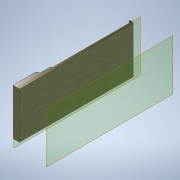
# Autodesk Inventor part: ShipDesign-ver3-1111-2021
Saved by Autodesk Inventor 2021 (Build 250183000, 183)
## iProperties
Created: 2021-02-04
Part Number: ShipDesign-ver3-1111-2021
Material: Wood (Oak)
Document SubType Name: Modeling
Designer: CMurray
Density: 0.76 g/cm^3
Appearance: Wood - Vertical White
Author: CMurray
Autodesk Inventor part; units mm, degrees
ref_plane "YZ Plane" through (0, 0, 0) normal (1, 0, 0) x (0, 1, 0)
ref_plane "XZ Plane" through (0, 0, 0) normal (0, 1, 0) x (-1, 0, 0)
ref_plane "XY Plane" through (0, 0, 0) normal (0, 0, 1) x (1, 0, 0)
sketch "Sketch1" plane through (0, 0, 0) normal (0, 1, 0) x (-1, 0, 0)
  line L0 (0, 0) -> (914.4, 0)
  line L1 (914.4, 0) -> (914.4, -70.0282)
  line L2 (0, 0) -> (508, 0)
  line L3 (914.4, 0) -> (660.4, 0)
  line L4 (660.4, 0) -> (611.4196, -58.3726)
  arc A0 (611.4196, -58.3726) -> (0, -274.3016) centre (714.4556, -1323.7323) ccw
  arc A1 (0, -2040.0836) -> (800.1, -3045.8561) centre (1469.1296, -1692.5086) ccw
  arc A2 (0, -274.3016) -> (0, -2040.0836) centre (7568.6791, -1157.1926) ccw
  line L5 (914.4, 0) -> (660.4, 0)
  line L6 (914.4, 0) -> (914.4, -635)
  line L7 (914.4, -635) -> (838.2, -635)
  line L8 (838.2, -635) -> (838.2, -939.8)
  line L9 (838.2, -939.8) -> (800.1, -939.8)
  line L10 (800.1, -939.8) -> (800.1, -3045.8561)
  dimension "d1" = 3048
  dimension "d2" = 508
  dimension "d11" = 76.2
  dimension "d12" = 130
  dimension "d14" = 7620
  dimension "d15" = 635
  dimension "d16" = 76.2
  dimension "d17" = 304.8
  dimension "d18" = 38.1
  constraints: 22 end point, 7 point on circle, 5 perpendicular, 3 centre point, 2 point on line, 1 collinear, 1 horizontal
  measures "d1" distance of L0.end L10.end
  measures "d2" distance of L0.start L2.end
  measures "d11" distance of L3.end L4.end
  measures "d12" angle of L0 L4
  measures "d14" radius of A2
  measures "d15" distance of L0.end L6.end
  measures "d16" distance of L6.end L7.end
  measures "d17" distance of L7.end L8.end
  measures "d18" distance of L8.end L9.end
extrude "Extrusion1" add sketch "Sketch1" along normal blind 1219.2
sketch "Sketch3" plane through (-914.4, 0, -635) normal (-1, 0, 0) x (0, 0, 1)
  line L0 (0, 0) -> (635, 0) projected
  line L1 (0, 0) -> (0, 1219.2) projected
  line L2 (635, 0) -> (0, 0)
  line L3 (0, 0) -> (0, 1219.2)
  line L4 (0, 1219.2) -> (635, 1219.2)
  line L5 (635, 1219.2) -> (635, 0)
  line L6 (584.2, 50.8) -> (50.8, 50.8)
  line L7 (50.8, 1168.4) -> (584.2, 1168.4)
  line L8 (584.2, 1168.4) -> (584.2, 50.8)
  line L9 (50.8, 50.8) -> (0, 50.8)
  line L10 (0, 0) -> (0, 1219.2) projected
  line L11 (0, 50.8) -> (0, 1168.4)
  line L12 (50.8, 1168.4) -> (0, 1168.4)
  point P0 (0, 1168.4)
  dimension "d24" = 50.8
  constraints: 20 end point, 3 parallel, 3 perpendicular, 2 point on line, 1 horizontal, 1 other
  measures "d24" distance between parallel lines of L5 L8
extrude "Extrusion3" cut sketch "Sketch3" against normal blind 50.8 contours L1 L12 L7 L8 L6 L9
sketch "Sketch4" plane through (-838.2, 0, -939.8) normal (-1, 0, 0) x (0, 0, 1)
  line L0 (0, 1219.2) -> (304.8, 1219.2) projected
  line L1 (304.8, 0) -> (0, 0)
  line L2 (0, 0) -> (0, 1219.2)
  line L3 (0, 1219.2) -> (304.8, 1219.2)
  line L4 (304.8, 1219.2) -> (304.8, 0)
  line L5 (254, 50.8) -> (50.8, 50.8)
  line L6 (50.8, 1168.4) -> (254, 1168.4)
  line L7 (50.8, 1168.4) -> (0, 1168.4)
  line L8 (0, 0) -> (0, 1219.2) projected
  line L9 (50.8, 50.8) -> (0, 50.8)
  line L10 (0, 50.8) -> (0, 1168.4)
  line L11 (254, 50.8) -> (304.8, 50.8)
  line L12 (304.8, 50.8) -> (304.8, 1168.4)
  line L13 (304.8, 0) -> (304.8, 1219.2) projected
  line L14 (254, 1168.4) -> (304.8, 1168.4)
  point P0 (939.8, 0)
  constraints: 24 end point, 5 perpendicular, 4 parallel, 4 point on line, 1 horizontal
extrude "Extrusion4" cut sketch "Sketch4" against normal blind 50.8 contours L7 L6 L14 L4 L11 L5 L9 L2
sketch "Sketch5" plane through (-800.1, 0, -3045.8561) normal (-1, 0, 0) x (0, 0, 1)
  line L0 (0, 1219.2) -> (2106.0561, 1219.2) projected
  line L1 (2106.0561, 0) -> (0, 0)
  line L2 (0, 0) -> (0, 1219.2)
  line L3 (0, 1219.2) -> (2106.0561, 1219.2)
  line L4 (2106.0561, 1219.2) -> (2106.0561, 0)
  line L5 (2055.2561, 50.8) -> (50.8, 50.8)
  line L6 (50.8, 50.8) -> (50.8, 1168.4)
  line L7 (50.8, 1168.4) -> (2055.2561, 1168.4)
  line L8 (2055.2561, 50.8) -> (2106.0561, 50.8)
  line L9 (2106.0561, 0) -> (2106.0561, 1219.2) projected
  line L10 (2106.0561, 1168.4) -> (2106.0561, 1219.2) projected
  line L11 (2055.2561, 1168.4) -> (2106.0561, 1168.4)
  line L12 (2106.0561, 1168.4) -> (2106.0561, 50.8)
  point P0 (3045.8561, 0)
  constraints: 20 end point, 3 horizontal, 3 parallel, 3 perpendicular, 1 point on line, 2 other
extrude "Extrusion5" cut sketch "Sketch5" against normal blind 50.8 contours L4 L8 L5 L6 L7 L11
sketch "Sketch6" plane through (-800.1, 0, -3045.8561) normal (-1, 0, 0) x (0, 0, 1)
  line L0 (0, 0) -> (0, 1219.2) projected
  line L1 (0, 0) -> (2106.0561, 0) projected
  line L2 (0, 1219.2) -> (50.8, 1219.2)
  line L3 (50.8, 1219.2) -> (50.8, 0)
  line L4 (50.8, 0) -> (0, 0)
  line L5 (0, 0) -> (0, 1219.2)
  point P0 (3045.8561, 0)
  dimension "d33" = 50.8
  constraints: 8 end point, 2 parallel, 1 horizontal, 1 perpendicular, 1 point on line
  measures "d33" distance between parallel lines of L3 L0
extrude "Extrusion6" add sketch "Sketch6" along normal blind 50.8
fillet "Fillet1" radius 25.4 1 edges at (-850.9, 609.6, -2995.0561)
fillet "Fillet2" radius 6.35 1 edges at (-850.9, 609.6, -3045.8561)
fillet "Fillet3" radius 12.7 1 edges at (-800.1, 609.6, -3045.8561)
fillet "Fillet4" radius 25.4 1 edges at (0, 609.6, -274.3016)
fillet "Fillet5" radius 57.15 1 edges at (-914.4, 1193.8, -635)
fillet "Fillet6" radius 57.15 1 edges at (-838.2, 1193.8, -939.8)
fillet "Fillet7" radius 6.35 1 edges at (-914.4, 609.6, 0)
ref_plane "Work Plane6" through (-736.6, 50.8, -50.8) normal (-1, 0, 0) x (0, 0, 1)
ref_plane "Work Plane7" through (128.5875, 50.8, -50.8) normal (-1, 0, 0) x (0, 0, 1)
sketch "Sketch9" plane through (128.5875, 50.8, -50.8) normal (-1, 0, 0) x (0, 0, 1)
  line L0 (204.9292, -115.2136) -> (-3165.499, -115.2136)
  line L1 (-3165.499, -115.2136) -> (-3165.499, 1233.5764)
  line L2 (-3165.499, 1233.5764) -> (204.9292, 1233.5764)
  line L3 (204.9292, 1233.5764) -> (204.9292, -115.2136)
  point P0 (50.8, -50.8)
  constraints: 8 end point, 2 parallel, 1 horizontal, 1 perpendicular
extrude "Extrusion7" cut sketch "Sketch9" along normal blind 865.2002
body "Solid1"
